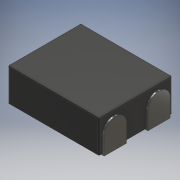
# Autodesk Inventor part: 4pin_smd
Saved by Autodesk Inventor 2020.3 (Build 243373000, 373)
## iProperties
Created: 2018-02-03
Part Number: 4pin_smd
Material: Genérico
Document SubType Name: Modeling
Designer: RafaX
Density: 1 g/cm^3
Appearance: Valor por defecto
Author: RafaX
Autodesk Inventor part; units mm, degrees
ref_plane "YZ Plane" through (0, 0, 0) normal (1, 0, 0) x (0, 1, 0)
ref_plane "XZ Plane" through (0, 0, 0) normal (0, 1, 0) x (-1, 0, 0)
ref_plane "XY Plane" through (0, 0, 0) normal (0, 0, 1) x (1, 0, 0)
sketch "Boceto1" plane through (0, 0, 0) normal (0, 0, 1) x (1, 0, 0)
  line L0 (-4.2825, 0.0488) -> (-3.0325, 0.0488)
  line L1 (-3.0325, 0.0488) -> (-3.0325, -0.9512)
  line L2 (-3.0325, -0.9512) -> (-4.2825, -0.9512)
  line L3 (-4.2825, -0.9512) -> (-4.2825, 0.0488)
  point P0 (0, 0)
  dimension "d0" = 1.25
  dimension "d1" = 1
  constraints: 8 end point, 2 parallel, 1 horizontal, 1 perpendicular
  measures "d0" distance of L1.end L2.end
  measures "d1" distance of L0.end L1.end
extrude "Extrusión1" add sketch "Boceto1" along normal blind 0.45
ref_plane "Plano de trabajo1" through (-4.2825, -0.9512, 0.45) normal (-1, 0, 0) x (0, -1, 0)
sketch "Boceto2" plane through (-4.2825, -0.9512, 0.45) normal (-1, 0, 0) x (0, -1, 0)
  line L0 (-0.9512, -0.45) -> (-0.6471, -0.45)
  line L1 (-0.6471, -0.45) -> (-0.6471, -0.2073)
  line L2 (-0.9512, -0.2073) -> (-0.9512, -0.45)
  arc A0 (-0.6471, -0.2219) -> (-0.9512, -0.2219) centre (-0.7992, -0.2073) ccw
  line L3 (0, -0.45) -> (-1, -0.45) projected
  line L4 (-0.0488, -0.45) -> (-0.3529, -0.45)
  line L5 (-0.3529, -0.45) -> (-0.3529, -0.2073)
  line L6 (-0.0488, -0.2073) -> (-0.0488, -0.45)
  arc A1 (-0.0488, -0.2219) -> (-0.3529, -0.2219) centre (-0.2008, -0.2073) ccw
  constraints: 12 end point, 4 point on circle, 4 point on line, 2 centre point, 1 horizontal, 1 parallel, 1 perpendicular
extrude "Extrusión2" add sketch "Boceto2" against normal blind 0.3 separate body
move or copy body "Desplazar1" bodies to move or copy 2 copy no translate (-0.02, 0, -0.02)
ref_plane "Plano de trabajo3" through (-3.6575, 0.0488, 0.45) normal (1, 0, 0) x (0, 1, 0)
ref_plane "Plano de trabajo2" through (-3.0325, 0.0488, 0.45) normal (1, 0, 0) x (0, 1, 0)
mirror "Simetría1" about plane through (-3.6575, 0.0488, 0.45) normal (1, 0, 0) bodies 2 separate body
fillet "Empalme1" radius 0.02 8 edges at (-4.2825, -0.4512, 0.45) (-3.6575, -0.9512, 0.45) (-3.0325, -0.4512, 0.45) (-3.0325, -0.9512, 0.225) (-4.2825, -0.9512, 0.225) (-4.2825, 0.0488, 0.225) (-3.6575, 0.0488, 0.45) (-3.0325, 0.0488, 0.225)
